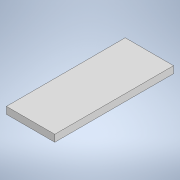
# Autodesk Inventor part: PCB
Saved by Autodesk Inventor 2021 (Build 250183000, 183)
## iProperties
Created: 2021-04-23
Part Number: PCB
Material: Ogólny
Document SubType Name: Modeling
Designer: jakub
Density: 1 g/cm^3
Appearance: Domyślna
Author: jakub
Autodesk Inventor part; units mm, degrees
ref_plane "YZ Plane" through (0, 0, 0) normal (1, 0, 0) x (0, 1, 0)
ref_plane "XZ Plane" through (0, 0, 0) normal (0, 1, 0) x (-1, 0, 0)
ref_plane "XY Plane" through (0, 0, 0) normal (0, 0, 1) x (1, 0, 0)
sketch "Szkic1" plane through (0, 0, 0) normal (0, 1, 0) x (-1, 0, 0)
  line L0 (0, 0) -> (-42, 0)
  line L1 (-42, 0) -> (-42, -86)
  line L2 (-42, -86) -> (0, -86)
  line L3 (0, -86) -> (0, 0)
  dimension "d0" = 42
  dimension "d1" = 86
  constraints: 8 end point, 2 parallel, 1 horizontal, 1 perpendicular
  measures "d0" distance of L2.end L1.end
  measures "d1" distance of L1.end L0.end
extrude "Wyciągnięcie proste1" add sketch "Szkic1" along normal blind 5
sketch "Szkic2" plane through (0, 0, 0) normal (0, 0, 1) x (1, 0, 0)
  line L0 (42, 0) -> (42, 5) projected
  line L1 (42, 5) -> (0, 5) projected
  line L2 (42, 0) -> (35, 0)
  line L3 (35, 0) -> (35, 5)
  line L4 (35, 5) -> (42, 5)
  line L5 (42, 5) -> (42, 0)
  point P0 (0, 0)
  dimension "d4" = 7
  constraints: 8 end point, 2 parallel, 1 horizontal, 1 perpendicular, 1 point on line
  measures "d4" distance of L3.end L4.end
extrude "Wyciągnięcie proste2" cut sketch "Szkic2" against normal blind 106.25
